Autodesk Inventor part; units mm, degrees
(part 2 of 7)
  line L845 (-272.2013, -12.84) -> (-271.8153, -13.0066)
  line L846 (-271.8153, -13.0066) -> (-271.4089, -13.1307)
  line L847 (-271.4089, -13.1307) -> (-270.9874, -13.2134)
  line L848 (-270.9874, -13.2134) -> (-270.5558, -13.2559)
  line L849 (-270.5558, -13.2559) -> (-270.1196, -13.2593)
  line L850 (-270.1196, -13.2593) -> (-269.6838, -13.2245)
  line L851 (-269.6838, -13.2245) -> (-269.2538, -13.1528)
  line L852 (-269.2538, -13.1528) -> (-268.8348, -13.0453)
  line L853 (-268.8348, -13.0453) -> (-268.4319, -12.9031)
  line L854 (-268.4319, -12.9031) -> (-268.0504, -12.7271)
  line L855 (-268.0504, -12.7271) -> (-267.6956, -12.5187)
  line L856 (-267.6956, -12.5187) -> (-267.3727, -12.2788)
  line L857 (-267.3727, -12.2788) -> (-267.0868, -12.0086)
  line L858 (-267.0868, -12.0086) -> (-266.8433, -11.7091)
  line L859 (-266.8433, -11.7091) -> (-266.6473, -11.3815)
  line L860 (-266.6473, -11.3815) -> (-266.462, -10.9873)
  line L861 (-266.462, -10.9873) -> (-266.3277, -10.6383)
  line L862 (-266.3277, -10.6383) -> (-266.2438, -10.3185)
  line L863 (-266.2438, -10.3185) -> (-266.2099, -10.0121)
  line L864 (-266.2099, -10.0121) -> (-266.2256, -9.703)
  line L865 (-266.2256, -9.703) -> (-266.2902, -9.3753)
  line L866 (-266.2902, -9.3753) -> (-266.4035, -9.013)
  line L867 (-266.4035, -9.013) -> (-266.5648, -8.6003)
  line L868 (-267.3452, -32.2865) -> (-267.8792, -32.2536)
  line L869 (-267.8792, -32.2536) -> (-268.3624, -32.1575)
  line L870 (-268.3624, -32.1575) -> (-268.7797, -32.0027)
  line L871 (-268.7797, -32.0027) -> (-269.116, -31.7932)
  line L872 (-269.116, -31.7932) -> (-269.7252, -31.2998)
  line L873 (-269.7252, -31.2998) -> (-267.9545, -30.2814)
  line L874 (-267.9545, -30.2814) -> (-267.6846, -30.1248)
  line L875 (-267.6846, -30.1248) -> (-267.4428, -29.9813)
  line L876 (-267.4428, -29.9813) -> (-267.2276, -29.8494)
  line L877 (-267.2276, -29.8494) -> (-267.0377, -29.7277)
  line L878 (-267.0377, -29.7277) -> (-266.7274, -29.5089)
  line L879 (-266.7274, -29.5089) -> (-266.5001, -29.3132)
  line L880 (-266.5001, -29.3132) -> (-266.3439, -29.1287)
  line L881 (-266.3439, -29.1287) -> (-266.2471, -28.9437)
  line L882 (-266.2471, -28.9437) -> (-266.1976, -28.7466)
  line L883 (-266.1976, -28.7466) -> (-266.1838, -28.5255)
  line L884 (-266.1838, -28.5255) -> (-266.1936, -28.2391)
  line L885 (-266.1936, -28.2391) -> (-266.2202, -28.0046)
  line L886 (-266.2202, -28.0046) -> (-266.2386, -27.9144)
  line L887 (-266.2386, -27.9144) -> (-266.2597, -27.8462)
  line L888 (-266.2597, -27.8462) -> (-266.283, -27.803)
  line L889 (-266.283, -27.803) -> (-266.308, -27.788)
  line L890 (-266.308, -27.788) -> (-266.379, -27.8152)
  line L891 (-266.379, -27.8152) -> (-266.5342, -27.8931)
  line L892 (-266.5342, -27.8931) -> (-266.7639, -28.0164)
  line L893 (-266.7639, -28.0164) -> (-267.0584, -28.1794)
  line L894 (-267.0584, -28.1794) -> (-267.4079, -28.3768)
  line L895 (-267.4079, -28.3768) -> (-267.8025, -28.6032)
  line L896 (-267.8025, -28.6032) -> (-268.2326, -28.8529)
  line L897 (-268.2326, -28.8529) -> (-268.6883, -29.1206)
  line L898 (-268.6883, -29.1206) -> (-270.9445, -30.4532)
  line L899 (-270.9445, -30.4532) -> (-272.359, -29.3852)
  line L900 (-272.359, -29.3852) -> (-272.6467, -29.1707)
  line L901 (-272.6467, -29.1707) -> (-272.922, -28.9705)
  line L902 (-272.922, -28.9705) -> (-273.1783, -28.7891)
  line L903 (-273.1783, -28.7891) -> (-273.4093, -28.6309)
  line L904 (-273.4093, -28.6309) -> (-273.6082, -28.5003)
  line L905 (-273.6082, -28.5003) -> (-273.7686, -28.4015)
  line L906 (-273.7686, -28.4015) -> (-273.884, -28.339)
  line L907 (-273.884, -28.339) -> (-273.948, -28.3172)
  line L908 (-273.948, -28.3172) -> (-274.0152, -28.3746)
  line L909 (-274.0152, -28.3746) -> (-274.0693, -28.531)
  line L910 (-274.0693, -28.531) -> (-274.1047, -28.7624)
  line L911 (-274.1047, -28.7624) -> (-274.116, -29.0449)
  line L912 (-274.116, -29.0449) -> (-274.099, -29.2561)
  line L913 (-274.099, -29.2561) -> (-274.0465, -29.4524)
  line L914 (-274.0465, -29.4524) -> (-273.9505, -29.6431)
  line L915 (-273.9505, -29.6431) -> (-273.8029, -29.8373)
  line L916 (-273.8029, -29.8373) -> (-273.5956, -30.0441)
  line L917 (-273.5956, -30.0441) -> (-273.3205, -30.2725)
  line L918 (-273.3205, -30.2725) -> (-272.9695, -30.5318)
  line L919 (-272.9695, -30.5318) -> (-272.5347, -30.8311)
  line L920 (-272.5347, -30.8311) -> (-272.2182, -31.0478)
  line L921 (-272.2182, -31.0478) -> (-271.9226, -31.2577)
  line L922 (-271.9226, -31.2577) -> (-271.6546, -31.4559)
  line L923 (-271.6546, -31.4559) -> (-271.4205, -31.6369)
  line L924 (-271.4205, -31.6369) -> (-271.2268, -31.7959)
  line L925 (-271.2268, -31.7959) -> (-271.0801, -31.9275)
  line L926 (-271.0801, -31.9275) -> (-270.9867, -32.0266)
  line L927 (-270.9867, -32.0266) -> (-270.9533, -32.088)
  line L928 (-270.9533, -32.088) -> (-270.9845, -32.1279)
  line L929 (-270.9845, -32.1279) -> (-271.0761, -32.1651)
  line L930 (-271.0761, -32.1651) -> (-271.2219, -32.1988)
  line L931 (-271.2219, -32.1988) -> (-271.4152, -32.2282)
  line L932 (-271.4152, -32.2282) -> (-271.6496, -32.2525)
  line L933 (-271.6496, -32.2525) -> (-271.9187, -32.2708)
  line L934 (-271.9187, -32.2708) -> (-272.2158, -32.2825)
  line L935 (-272.2158, -32.2825) -> (-272.5347, -32.2865)
  line L936 (-272.5347, -32.2865) -> (-274.1224, -32.2865)
  line L937 (-274.1224, -32.2865) -> (-274.1224, -33.0804)
  line L938 (-274.1224, -33.0804) -> (-274.1224, -33.8742)
  line L939 (-274.1224, -33.8742) -> (-270.1531, -33.8742)
  line L940 (-270.1531, -33.8742) -> (-266.1838, -33.8742)
  line L941 (-266.1838, -33.8742) -> (-266.1838, -33.0804)
  line L942 (-266.1838, -33.0804) -> (-266.188, -32.8276)
  line L943 (-266.188, -32.8276) -> (-266.2086, -32.6351)
  line L944 (-266.2086, -32.6351) -> (-266.2575, -32.4945)
  line L945 (-266.2575, -32.4945) -> (-266.3467, -32.3979)
  line L946 (-266.3467, -32.3979) -> (-266.4881, -32.3369)
  line L947 (-266.4881, -32.3369) -> (-266.6937, -32.3035)
  line L948 (-266.6937, -32.3035) -> (-266.9755, -32.2894)
  line L949 (-266.9755, -32.2894) -> (-267.3452, -32.2865)
  line L950 (-270.1531, 32.2808) -> (-274.1224, 32.2808)
  line L951 (-274.1224, 32.2808) -> (-274.1224, 31.6192)
  line L952 (-274.1224, 31.6192) -> (-274.1224, 30.9577)
  line L953 (-274.1224, 30.9577) -> (-270.1531, 30.9577)
  line L954 (-270.1531, 30.9577) -> (-266.1838, 30.9577)
  line L955 (-266.1838, 30.9577) -> (-266.1838, 31.6192)
  line L956 (-266.1838, 31.6192) -> (-266.1838, 32.2808)
  line L957 (-266.1838, 32.2808) -> (-270.1531, 32.2808)
  line L958 (-267.6392, -18.7909) -> (-267.8826, -18.7903)
  line L959 (-267.8826, -18.7903) -> (-268.0973, -18.7881)
  line L960 (-268.0973, -18.7881) -> (-268.2851, -18.7835)
  line L961 (-268.2851, -18.7835) -> (-268.4478, -18.7755)
  line L962 (-268.4478, -18.7755) -> (-268.7051, -18.7465)
  line L963 (-268.7051, -18.7465) -> (-268.8835, -18.6945)
  line L964 (-268.8835, -18.6945) -> (-268.9974, -18.6131)
  line L965 (-268.9974, -18.6131) -> (-269.0609, -18.4956)
  line L966 (-269.0609, -18.4956) -> (-269.0886, -18.3356)
  line L967 (-269.0886, -18.3356) -> (-269.0946, -18.1265)
  line L968 (-269.0946, -18.1265) -> (-269.0808, -17.9354)
  line L969 (-269.0808, -17.9354) -> (-269.0343, -17.7642)
  line L970 (-269.0343, -17.7642) -> (-268.9474, -17.6057)
  line L971 (-268.9474, -17.6057) -> (-268.8125, -17.4525)
  line L972 (-268.8125, -17.4525) -> (-268.6218, -17.2974)
  line L973 (-268.6218, -17.2974) -> (-268.3679, -17.1332)
  line L974 (-268.3679, -17.1332) -> (-268.0429, -16.9525)
  line L975 (-268.0429, -16.9525) -> (-267.6392, -16.7482)
  line L976 (-267.6392, -16.7482) -> (-267.4074, -16.6334)
  line L977 (-267.4074, -16.6334) -> (-267.2014, -16.5284)
  line L978 (-267.2014, -16.5284) -> (-267.0195, -16.4315)
  line L979 (-267.0195, -16.4315) -> (-266.8603, -16.3412)
  line L980 (-266.8603, -16.3412) -> (-266.6043, -16.174)
  line L981 (-266.6043, -16.174) -> (-266.4213, -16.0143)
  line L982 (-266.4213, -16.0143) -> (-266.2996, -15.8493)
  line L983 (-266.2996, -15.8493) -> (-266.2274, -15.6666)
  line L984 (-266.2274, -15.6666) -> (-266.1927, -15.4534)
  line L985 (-266.1927, -15.4534) -> (-266.1838, -15.1971)
  line L986 (-266.1838, -15.1971) -> (-266.1838, -14.3597)
  line L987 (-266.1838, -14.3597) -> (-267.7535, -15.1829)
  line L988 (-267.7535, -15.1829) -> (-269.3232, -16.0061)
  line L989 (-269.3232, -16.0061) -> (-269.9537, -15.4139)
  line L990 (-269.9537, -15.4139) -> (-270.247, -15.1962)
  line L991 (-270.247, -15.1962) -> (-270.6031, -15.0254)
  line L992 (-270.6031, -15.0254) -> (-271.0044, -14.9035)
  line L993 (-271.0044, -14.9035) -> (-271.4332, -14.8321)
  line L994 (-271.4332, -14.8321) -> (-271.8718, -14.8131)
  line L995 (-271.8718, -14.8131) -> (-272.3025, -14.8485)
  line L996 (-272.3025, -14.8485) -> (-272.7077, -14.9399)
  line L997 (-272.7077, -14.9399) -> (-273.0697, -15.0893)
  line L998 (-273.0697, -15.0893) -> (-273.1839, -15.1649)
  line L999 (-273.1839, -15.1649) -> (-273.2933, -15.2662)
  line L1000 (-273.2933, -15.2662) -> (-273.3974, -15.3921)
  line L1001 (-273.3974, -15.3921) -> (-273.496, -15.5412)
  line L1002 (-273.496, -15.5412) -> (-273.675, -15.9049)
  line L1003 (-273.675, -15.9049) -> (-273.8277, -16.3478)
  line L1004 (-273.8277, -16.3478) -> (-273.9514, -16.8606)
  line L1005 (-273.9514, -16.8606) -> (-274.0433, -17.434)
  line L1006 (-274.0433, -17.434) -> (-274.1007, -18.0585)
  line L1007 (-274.1007, -18.0585) -> (-274.1209, -18.7247)
  line L1008 (-274.1209, -18.7247) -> (-274.1224, -20.114)
  line L1009 (-274.1224, -20.114) -> (-270.1531, -20.114)
  line L1010 (-270.1531, -20.114) -> (-266.1838, -20.114)
  line L1011 (-266.1838, -20.114) -> (-266.1838, -19.4524)
  line L1012 (-266.1838, -19.4524) -> (-266.1899, -19.2444)
  line L1013 (-266.1899, -19.2444) -> (-266.2177, -19.0852)
  line L1014 (-266.2177, -19.0852) -> (-266.2814, -18.9683)
  line L1015 (-266.2814, -18.9683) -> (-266.3955, -18.8871)
  line L1016 (-266.3955, -18.8871) -> (-266.574, -18.8353)
  line L1017 (-266.574, -18.8353) -> (-266.8313, -18.8063)
  line L1018 (-266.8313, -18.8063) -> (-266.9939, -18.7983)
  line L1019 (-266.9939, -18.7983) -> (-267.1816, -18.7937)
  line L1020 (-267.1816, -18.7937) -> (-267.3961, -18.7914)
  line L1021 (-267.3961, -18.7914) -> (-267.6392, -18.7909)
  line L1022 (-266.9776, 6.348) -> (-267.7715, 6.348)
  line L1023 (-267.7715, 6.348) -> (-267.7715, 4.628)
  line L1024 (-267.7715, 4.628) -> (-267.7715, 2.9079)
  line L1025 (-267.7715, 2.9079) -> (-268.6977, 2.9079)
  line L1026 (-268.6977, 2.9079) -> (-269.6238, 2.9079)
  line L1027 (-269.6238, 2.9079) -> (-269.6238, 4.2311)
  line L1028 (-269.6238, 4.2311) -> (-269.6269, 4.6425)
  line L1029 (-269.6269, 4.6425) -> (-269.6404, 4.9588)
  line L1030 (-269.6404, 4.9588) -> (-269.6703, 5.1924)
  line L1031 (-269.6703, 5.1924) -> (-269.7231, 5.3557)
  line L1032 (-269.7231, 5.3557) -> (-269.8047, 5.4611)
  line L1033 (-269.8047, 5.4611) -> (-269.9215, 5.5211)
  line L1034 (-269.9215, 5.5211) -> (-270.0797, 5.5479)
  line L1035 (-270.0797, 5.5479) -> (-270.2854, 5.5542)
  line L1036 (-270.2854, 5.5542) -> (-270.4911, 5.5479)
  line L1037 (-270.4911, 5.5479) -> (-270.6492, 5.5211)
  line L1038 (-270.6492, 5.5211) -> (-270.766, 5.4611)
  line L1039 (-270.766, 5.4611) -> (-270.8477, 5.3557)
  line L1040 (-270.8477, 5.3557) -> (-270.9004, 5.1924)
  line L1041 (-270.9004, 5.1924) -> (-270.9304, 4.9588)
  line L1042 (-270.9304, 4.9588) -> (-270.9438, 4.6425)
  line L1043 (-270.9438, 4.6425) -> (-270.9469, 4.2311)
  line L1044 (-270.9469, 4.2311) -> (-270.9473, 4.003)
  line L1045 (-270.9473, 4.003) -> (-270.9492, 3.8028)
  line L1046 (-270.9492, 3.8028) -> (-270.9537, 3.6285)
  line L1047 (-270.9537, 3.6285) -> (-270.9618, 3.4785)
  line L1048 (-270.9618, 3.4785) -> (-270.9935, 3.2439)
  line L1049 (-270.9935, 3.2439) -> (-271.0528, 3.0844)
  line L1050 (-271.0528, 3.0844) -> (-271.1485, 2.9855)
  line L1051 (-271.1485, 2.9855) -> (-271.2893, 2.9328)
  line L1052 (-271.2893, 2.9328) -> (-271.4838, 2.9117)
  line L1053 (-271.4838, 2.9117) -> (-271.7408, 2.9079)
  line L1054 (-271.7408, 2.9079) -> (-272.5347, 2.9079)
  line L1055 (-272.5347, 2.9079) -> (-272.5347, 4.4957)
  line L1056 (-272.5347, 4.4957) -> (-272.5347, 6.0834)
  line L1057 (-272.5347, 6.0834) -> (-273.3285, 6.0834)
  line L1058 (-273.3285, 6.0834) -> (-274.1224, 6.0834)
  line L1059 (-274.1224, 6.0834) -> (-274.1224, 3.8341)
  line L1060 (-274.1224, 3.8341) -> (-274.1224, 1.5849)
  line L1061 (-274.1224, 1.5849) -> (-270.1531, 1.5849)
  line L1062 (-270.1531, 1.5849) -> (-266.1838, 1.5849)
  line L1063 (-266.1838, 1.5849) -> (-266.1838, 3.9664)
  line L1064 (-266.1838, 3.9664) -> (-266.1838, 6.348)
  line L1065 (-266.1838, 6.348) -> (-266.9776, 6.348)
  line L1066 (-271.4762, -18.7909) -> (-272.5651, -18.7909)
  line L1067 (-272.5651, -18.7909) -> (-272.4837, -17.6932)
  line L1068 (-272.4837, -17.6932) -> (-272.4371, -17.3233)
  line L1069 (-272.4371, -17.3233) -> (-272.3587, -17.0028)
  line L1070 (-272.3587, -17.0028) -> (-272.2532, -16.7315)
  line L1071 (-272.2532, -16.7315) -> (-272.125, -16.5096)
  line L1072 (-272.125, -16.5096) -> (-271.9786, -16.337)
  line L1073 (-271.9786, -16.337) -> (-271.8187, -16.2137)
  line L1074 (-271.8187, -16.2137) -> (-271.6497, -16.1397)
  line L1075 (-271.6497, -16.1397) -> (-271.4762, -16.1151)
  line L1076 (-271.4762, -16.1151) -> (-271.3026, -16.1397)
  line L1077 (-271.3026, -16.1397) -> (-271.1336, -16.2137)
  line L1078 (-271.1336, -16.2137) -> (-270.9737, -16.337)
  line L1079 (-270.9737, -16.337) -> (-270.8273, -16.5096)
  line L1080 (-270.8273, -16.5096) -> (-270.6991, -16.7315)
  line L1081 (-270.6991, -16.7315) -> (-270.5936, -17.0028)
  line L1082 (-270.5936, -17.0028) -> (-270.5152, -17.3233)
  line L1083 (-270.5152, -17.3233) -> (-270.4686, -17.6932)
  line L1084 (-270.4686, -17.6932) -> (-270.3873, -18.7909)
  line L1085 (-270.3873, -18.7909) -> (-271.4762, -18.7909)
  line L1086 (-269.3592, -23.8187) -> (-272.5347, -23.8187)
  line L1087 (-272.5347, -23.8187) -> (-272.5347, -22.7602)
  line L1088 (-272.5347, -22.7602) -> (-272.538, -22.4277)
  line L1089 (-272.538, -22.4277) -> (-272.5533, -22.1731)
  line L1090 (-272.5533, -22.1731) -> (-272.5882, -21.986)
  line L1091 (-272.5882, -21.986) -> (-272.6504, -21.8561)
  line L1092 (-272.6504, -21.8561) -> (-272.7478, -21.773)
  line L1093 (-272.7478, -21.773) -> (-272.8882, -21.7265)
  line L1094 (-272.8882, -21.7265) -> (-273.0791, -21.7062)
  line L1095 (-273.0791, -21.7062) -> (-273.3285, -21.7017)
  line L1096 (-273.3285, -21.7017) -> (-274.1224, -21.7017)
  line L1097 (-274.1224, -21.7017) -> (-274.1224, -24.6125)
  line L1098 (-274.1224, -24.6125) -> (-274.1224, -27.5233)
  line L1099 (-274.1224, -27.5233) -> (-273.3285, -27.5233)
  line L1100 (-273.3285, -27.5233) -> (-273.0791, -27.5189)
  line L1101 (-273.0791, -27.5189) -> (-272.8882, -27.4985)
  line L1102 (-272.8882, -27.4985) -> (-272.7478, -27.452)
  line L1103 (-272.7478, -27.452) -> (-272.6504, -27.369)
  line L1104 (-272.6504, -27.369) -> (-272.5882, -27.2391)
  line L1105 (-272.5882, -27.2391) -> (-272.5533, -27.052)
  line L1106 (-272.5533, -27.052) -> (-272.538, -26.7974)
  line L1107 (-272.538, -26.7974) -> (-272.5347, -26.4649)
  line L1108 (-272.5347, -26.4649) -> (-272.5347, -25.4064)
  line L1109 (-272.5347, -25.4064) -> (-269.3592, -25.4064)
  line L1110 (-269.3592, -25.4064) -> (-266.1838, -25.4064)
  line L1111 (-266.1838, -25.4064) -> (-266.1838, -24.6125)
  line L1112 (-266.1838, -24.6125) -> (-266.1838, -23.8187)
  line L1113 (-266.1838, -23.8187) -> (-269.3592, -23.8187)
  line L1114 (-267.2516, 35.9855) -> (-267.6695, 36.0151)
  line L1115 (-267.6695, 36.0151) -> (-268.0934, 36.0965)
  line L1116 (-268.0934, 36.0965) -> (-268.5004, 36.2188)
  line L1117 (-268.5004, 36.2188) -> (-268.8676, 36.3711)
  line L1118 (-268.8676, 36.3711) -> (-269.1723, 36.5421)
  line L1119 (-269.1723, 36.5421) -> (-269.3916, 36.7211)
  line L1120 (-269.3916, 36.7211) -> (-269.462, 36.8101)
  line L1121 (-269.462, 36.8101) -> (-269.5025, 36.897)
  line L1122 (-269.5025, 36.897) -> (-269.5103, 36.9803)
  line L1123 (-269.5103, 36.9803) -> (-269.4824, 37.0588)
  line L1124 (-269.4824, 37.0588) -> (-269.4226, 37.121)
  line L1125 (-269.4226, 37.121) -> (-269.3045, 37.2133)
  line L1126 (-269.3045, 37.2133) -> (-269.135, 37.3313)
  line L1127 (-269.135, 37.3313) -> (-268.9213, 37.4705)
  line L1128 (-268.9213, 37.4705) -> (-268.3892, 37.7944)
  line L1129 (-268.3892, 37.7944) -> (-267.7646, 38.1494)
  line L1130 (-267.7646, 38.1494) -> (-267.3115, 38.4045)
  line L1131 (-267.3115, 38.4045) -> (-266.9516, 38.6234)
  line L1132 (-266.9516, 38.6234) -> (-266.6749, 38.8163)
  line L1133 (-266.6749, 38.8163) -> (-266.4711, 38.9937)
  line L1134 (-266.4711, 38.9937) -> (-266.3302, 39.1656)
  line L1135 (-266.3302, 39.1656) -> (-266.2421, 39.3423)
  line L1136 (-266.2421, 39.3423) -> (-266.1967, 39.5341)
  line L1137 (-266.1967, 39.5341) -> (-266.1838, 39.7512)
  line L1138 (-266.1838, 39.7512) -> (-266.1963, 40.0357)
  line L1139 (-266.1963, 40.0357) -> (-266.2303, 40.2687)
  line L1140 (-266.2303, 40.2687) -> (-266.2538, 40.3584)
  line L1141 (-266.2538, 40.3584) -> (-266.2807, 40.4262)
  line L1142 (-266.2807, 40.4262) -> (-266.3104, 40.469)
  line L1143 (-266.3104, 40.469) -> (-266.3422, 40.484)
  line L1144 (-266.3422, 40.484) -> (-266.4193, 40.4574)
  line L1145 (-266.4193, 40.4574) -> (-266.5788, 40.381)
  line L1146 (-266.5788, 40.381) -> (-266.8108, 40.2603)
  line L1147 (-266.8108, 40.2603) -> (-267.1057, 40.1005)
  line L1148 (-267.1057, 40.1005) -> (-267.4536, 39.9071)
  line L1149 (-267.4536, 39.9071) -> (-267.845, 39.6854)
  line L1150 (-267.845, 39.6854) -> (-268.2699, 39.4408)
  line L1151 (-268.2699, 39.4408) -> (-268.7187, 39.1785)
  line L1152 (-268.7187, 39.1785) -> (-270.9367, 37.8731)
  line L1153 (-270.9367, 37.8731) -> (-272.5295, 39.0457)
  line L1154 (-272.5295, 39.0457) -> (-274.1224, 40.2183)
  line L1155 (-274.1224, 40.2183) -> (-274.1224, 39.4243)
  line L1156 (-274.1224, 39.4243) -> (-274.109, 39.1889)
  line L1157 (-274.109, 39.1889) -> (-274.0625, 38.9758)
  line L1158 (-274.0625, 38.9758) -> (-273.973, 38.7732)
  line L1159 (-273.973, 38.7732) -> (-273.8309, 38.5695)
  line L1160 (-273.8309, 38.5695) -> (-273.6264, 38.3527)
  line L1161 (-273.6264, 38.3527) -> (-273.3499, 38.1111)
  line L1162 (-273.3499, 38.1111) -> (-273.1815, 37.9773)
  line L1163 (-273.1815, 37.9773) -> (-272.9915, 37.8329)
  line L1164 (-272.9915, 37.8329) -> (-272.7787, 37.6764)
  line L1165 (-272.7787, 37.6764) -> (-272.5417, 37.5064)
  line L1166 (-272.5417, 37.5064) -> (-272.224, 37.2765)
  line L1167 (-272.224, 37.2765) -> (-271.9274, 37.0543)
  line L1168 (-271.9274, 37.0543) -> (-271.6583, 36.8451)
  line L1169 (-271.6583, 36.8451) -> (-271.4233, 36.6543)
  line L1170 (-271.4233, 36.6543) -> (-271.2288, 36.4873)
  line L1171 (-271.2288, 36.4873) -> (-271.0814, 36.3497)
  line L1172 (-271.0814, 36.3497) -> (-270.9877, 36.2467)
  line L1173 (-270.9877, 36.2467) -> (-270.954, 36.1839)
  line L1174 (-270.954, 36.1839) -> (-270.985, 36.1441)
  line L1175 (-270.985, 36.1441) -> (-271.0765, 36.1069)
  line L1176 (-271.0765, 36.1069) -> (-271.2222, 36.0732)
  line L1177 (-271.2222, 36.0732) -> (-271.4154, 36.0438)
  line L1178 (-271.4154, 36.0438) -> (-271.6497, 36.0195)
  line L1179 (-271.6497, 36.0195) -> (-271.9187, 36.0011)
  line L1180 (-271.9187, 36.0011) -> (-272.2159, 35.9895)
  line L1181 (-272.2159, 35.9895) -> (-272.5347, 35.9855)
  line L1182 (-272.5347, 35.9855) -> (-274.1224, 35.9855)
  line L1183 (-274.1224, 35.9855) -> (-274.1224, 35.1916)
  line L1184 (-274.1224, 35.1916) -> (-274.1224, 34.3977)
  line L1185 (-274.1224, 34.3977) -> (-270.1531, 34.3977)
  line L1186 (-270.1531, 34.3977) -> (-266.1838, 34.3977)
  line L1187 (-266.1838, 34.3977) -> (-266.1838, 35.1916)
  line L1188 (-266.1838, 35.1916) -> (-266.1882, 35.4413)
  line L1189 (-266.1882, 35.4413) -> (-266.2086, 35.6324)
  line L1190 (-266.2086, 35.6324) -> (-266.2553, 35.7728)
  line L1191 (-266.2553, 35.7728) -> (-266.3389, 35.8701)
  line L1192 (-266.3389, 35.8701) -> (-266.4698, 35.9323)
  line L1193 (-266.4698, 35.9323) -> (-266.6586, 35.967)
  line L1194 (-266.6586, 35.967) -> (-266.9157, 35.9822)
  line L1195 (-266.9157, 35.9822) -> (-267.2516, 35.9855)
  line L1196 (-268.9628, 24.2931) -> (-269.5211, 24.2796)
  line L1197 (-269.5211, 24.2796) -> (-270.0419, 24.2734)
  line L1198 (-270.0419, 24.2734) -> (-270.5137, 24.274)
  line L1199 (-270.5137, 24.274) -> (-270.9254, 24.2813)
  line L1200 (-270.9254, 24.2813) -> (-271.2654, 24.2948)
  line L1201 (-271.2654, 24.2948) -> (-271.5223, 24.3143)
  line L1202 (-271.5223, 24.3143) -> (-271.616, 24.3262)
  line L1203 (-271.616, 24.3262) -> (-271.6847, 24.3394)
  line L1204 (-271.6847, 24.3394) -> (-271.727, 24.354)
  line L1205 (-271.727, 24.354) -> (-271.7413, 24.3698)
  line L1206 (-271.7413, 24.3698) -> (-271.7269, 24.3931)
  line L1207 (-271.7269, 24.3931) -> (-271.6845, 24.4296)
  line L1208 (-271.6845, 24.4296) -> (-271.6157, 24.4783)
  line L1209 (-271.6157, 24.4783) -> (-271.5219, 24.5386)
  line L1210 (-271.5219, 24.5386) -> (-271.2648, 24.6907)
  line L1211 (-271.2648, 24.6907) -> (-270.9248, 24.8797)
  line L1212 (-270.9248, 24.8797) -> (-270.5131, 25.0994)
  line L1213 (-270.5131, 25.0994) -> (-270.0412, 25.3436)
  line L1214 (-270.0412, 25.3436) -> (-269.5204, 25.6061)
  line L1215 (-269.5204, 25.6061) -> (-268.9623, 25.8807)
  line L1216 (-268.9623, 25.8807) -> (-268.4989, 26.1067)
  line L1217 (-268.4989, 26.1067) -> (-268.0899, 26.3083)
  line L1218 (-268.0899, 26.3083) -> (-267.7319, 26.4881)
  line L1219 (-267.7319, 26.4881) -> (-267.4216, 26.6487)
  line L1220 (-267.4216, 26.6487) -> (-267.1557, 26.7927)
  line L1221 (-267.1557, 26.7927) -> (-266.9305, 26.9229)
  line L1222 (-266.9305, 26.9229) -> (-266.743, 27.0417)
  line L1223 (-266.743, 27.0417) -> (-266.5895, 27.1519)
  line L1224 (-266.5895, 27.1519) -> (-266.3714, 27.3567)
  line L1225 (-266.3714, 27.3567) -> (-266.2491, 27.5583)
  line L1226 (-266.2491, 27.5583) -> (-266.1956, 27.7778)
  line L1227 (-266.1956, 27.7778) -> (-266.1838, 28.0362)
  line L1228 (-266.1838, 28.0362) -> (-266.1838, 28.8407)
  line L1229 (-266.1838, 28.8407) -> (-270.1531, 28.8407)
  line L1230 (-270.1531, 28.8407) -> (-274.1224, 28.8407)
  line L1231 (-274.1224, 28.8407) -> (-274.1224, 28.1792)
  line L1232 (-274.1224, 28.1792) -> (-274.1224, 27.5176)
  line L1233 (-274.1224, 27.5176) -> (-271.1454, 27.5148)
  line L1234 (-271.1454, 27.5148) -> (-268.1684, 27.512)
  line L1235 (-268.1684, 27.512) -> (-271.1454, 26.0402)
  line L1236 (-271.1454, 26.0402) -> (-271.6369, 25.7964)
  line L1237 (-271.6369, 25.7964) -> (-272.0714, 25.5788)
  line L1238 (-272.0714, 25.5788) -> (-272.4523, 25.3845)
  line L1239 (-272.4523, 25.3845) -> (-272.7832, 25.2111)
  line L1240 (-272.7832, 25.2111) -> (-273.0676, 25.0559)
  line L1241 (-273.0676, 25.0559) -> (-273.3089, 24.9162)
  line L1242 (-273.3089, 24.9162) -> (-273.5106, 24.7894)
  line L1243 (-273.5106, 24.7894) -> (-273.6763, 24.6728)
  line L1244 (-273.6763, 24.6728) -> (-273.8094, 24.5639)
  line L1245 (-273.8094, 24.5639) -> (-273.9134, 24.46)
  line L1246 (-273.9134, 24.46) -> (-273.9918, 24.3585)
  line L1247 (-273.9918, 24.3585) -> (-274.0481, 24.2566)
  line L1248 (-274.0481, 24.2566) -> (-274.1085, 24.0416)
  line L1249 (-274.1085, 24.0416) -> (-274.1224, 23.7937)
  line L1250 (-274.1224, 23.7937) -> (-274.1224, 23.0191)
  line L1251 (-274.1224, 23.0191) -> (-270.1531, 23.0191)
  line L1252 (-270.1531, 23.0191) -> (-266.1838, 23.0191)
  line L1253 (-266.1838, 23.0191) -> (-266.1838, 23.6977)
  line L1254 (-266.1838, 23.6977) -> (-266.1838, 24.3762)
  line L1255 (-266.1838, 24.3762) -> (-268.9628, 24.2931)
  line L1256 (-266.5537, 12.2782) -> (-266.7195, 12.653)
  line L1257 (-266.7195, 12.653) -> (-266.8708, 12.9403)
  line L1258 (-266.8708, 12.9403) -> (-267.0151, 13.1443)
  line L1259 (-267.0151, 13.1443) -> (-267.1598, 13.2696)
  line L1260 (-267.1598, 13.2696) -> (-267.3124, 13.3205)
  line L1261 (-267.3124, 13.3205) -> (-267.4805, 13.3015)
  line L1262 (-267.4805, 13.3015) -> (-267.6713, 13.2169)
  line L1263 (-267.6713, 13.2169) -> (-267.8925, 13.0714)
  line L1264 (-267.8925, 13.0714) -> (-268.0251, 12.9683)
  line L1265 (-268.0251, 12.9683) -> (-268.1253, 12.8753)
  line L1266 (-268.1253, 12.8753) -> (-268.1938, 12.7898)
  line L1267 (-268.1938, 12.7898) -> (-268.2314, 12.709)
  line L1268 (-268.2314, 12.709) -> (-268.2389, 12.6303)
  line L1269 (-268.2389, 12.6303) -> (-268.217, 12.5511)
  line L1270 (-268.217, 12.5511) -> (-268.1665, 12.4687)
  line L1271 (-268.1665, 12.4687) -> (-268.088, 12.3804)
  line L1272 (-268.088, 12.3804) -> (-267.9277, 12.1543)
  line L1273 (-267.9277, 12.1543) -> (-267.8259, 11.8684)
  line L1274 (-267.8259, 11.8684) -> (-267.7811, 11.54)
  line L1275 (-267.7811, 11.54) -> (-267.7913, 11.1865)
  line L1276 (-267.7913, 11.1865) -> (-267.8548, 10.8255)
  line L1277 (-267.8548, 10.8255) -> (-267.9697, 10.4744)
  line L1278 (-267.9697, 10.4744) -> (-268.1344, 10.1505)
  line L1279 (-268.1344, 10.1505) -> (-268.3468, 9.8713)
  line L1280 (-268.3468, 9.8713) -> (-268.5006, 9.7285)
  line L1281 (-268.5006, 9.7285) -> (-268.6748, 9.604)
  line L1282 (-268.6748, 9.604) -> (-268.8669, 9.4978)
  line L1283 (-268.8669, 9.4978) -> (-269.0743, 9.41)
  line L1284 (-269.0743, 9.41) -> (-269.525, 9.2898)
  line L1285 (-269.525, 9.2898) -> (-270.0066, 9.2436)
  line L1286 (-270.0066, 9.2436) -> (-270.4989, 9.2719)
  line L1287 (-270.4989, 9.2719) -> (-270.9817, 9.375)
  line L1288 (-270.9817, 9.375) -> (-271.4346, 9.5534)
  line L1289 (-271.4346, 9.5534) -> (-271.8374, 9.8073)
  line L1290 (-271.8374, 9.8073) -> (-272.0919, 10.0621)
  line L1291 (-272.0919, 10.0621) -> (-272.2942, 10.3738)
  line L1292 (-272.2942, 10.3738) -> (-272.4413, 10.7231)
  line L1293 (-272.4413, 10.7231) -> (-272.5302, 11.0907)
  line L1294 (-272.5302, 11.0907) -> (-272.5577, 11.4573)
  line L1295 (-272.5577, 11.4573) -> (-272.5209, 11.8033)
  line L1296 (-272.5209, 11.8033) -> (-272.4165, 12.1096)
  line L1297 (-272.4165, 12.1096) -> (-272.2416, 12.3568)
  line L1298 (-272.2416, 12.3568) -> (-272.1748, 12.4349)
  line L1299 (-272.1748, 12.4349) -> (-272.1355, 12.5091)
  line L1300 (-272.1355, 12.5091) -> (-272.1243, 12.581)
  line L1301 (-272.1243, 12.581) -> (-272.1419, 12.6517)
  line L1302 (-272.1419, 12.6517) -> (-272.1888, 12.7228)
  line L1303 (-272.1888, 12.7228) -> (-272.2656, 12.7955)
  line L1304 (-272.2656, 12.7955) -> (-272.3731, 12.8712)
  line L1305 (-272.3731, 12.8712) -> (-272.5117, 12.9512)
  line L1306 (-272.5117, 12.9512) -> (-272.7683, 13.0712)
  line L1307 (-272.7683, 13.0712) -> (-272.987, 13.1303)
  line L1308 (-272.987, 13.1303) -> (-273.1745, 13.1235)
  line L1309 (-273.1745, 13.1235) -> (-273.3378, 13.0455)
  line L1310 (-273.3378, 13.0455) -> (-273.4836, 12.8913)
  line L1311 (-273.4836, 12.8913) -> (-273.6188, 12.6557)
  line L1312 (-273.6188, 12.6557) -> (-273.7502, 12.3335)
  line L1313 (-273.7502, 12.3335) -> (-273.8846, 11.9198)
  line L1314 (-273.8846, 11.9198) -> (-273.9688, 11.6175)
  line L1315 (-273.9688, 11.6175) -> (-274.0247, 11.356)
  line L1316 (-274.0247, 11.356) -> (-274.0509, 11.1219)
  line L1317 (-274.0509, 11.1219) -> (-274.0462, 10.9019)
  line L1318 (-274.0462, 10.9019) -> (-274.0094, 10.6828)
  line L1319 (-274.0094, 10.6828) -> (-273.9391, 10.4511)
  line L1320 (-273.9391, 10.4511) -> (-273.8342, 10.1937)
  line L1321 (-273.8342, 10.1937) -> (-273.6934, 9.8972)
  line L1322 (-273.6934, 9.8972) -> (-273.3978, 9.3671)
  line L1323 (-273.3978, 9.3671) -> (-273.0765, 8.9234)
  line L1324 (-273.0765, 8.9234) -> (-272.7213, 8.5612)
  line L1325 (-272.7213, 8.5612) -> (-272.3242, 8.2755)
  line L1326 (-272.3242, 8.2755) -> (-271.8769, 8.0618)
  line L1327 (-271.8769, 8.0618) -> (-271.3714, 7.915)
  line L1328 (-271.3714, 7.915) -> (-270.7995, 7.8305)
  line L1329 (-270.7995, 7.8305) -> (-270.1531, 7.8034)
  line L1330 (-270.1531, 7.8034) -> (-269.5173, 7.8301)
  line L1331 (-269.5173, 7.8301) -> (-268.9518, 7.9129)
  line L1332 (-268.9518, 7.9129) -> (-268.4496, 8.0556)
  line L1333 (-268.4496, 8.0556) -> (-268.0038, 8.2623)
  line L1334 (-268.0038, 8.2623) -> (-267.6076, 8.5368)
  line L1335 (-267.6076, 8.5368) -> (-267.254, 8.8831)
  line L1336 (-267.254, 8.8831) -> (-266.9362, 9.3052)
  line L1337 (-266.9362, 9.3052) -> (-266.6473, 9.8069)
  line L1338 (-266.6473, 9.8069) -> (-266.4632, 10.1814)
  line L1339 (-266.4632, 10.1814) -> (-266.3299, 10.496)
  line L1340 (-266.3299, 10.496) -> (-266.2467, 10.7712)
  line L1341 (-266.2467, 10.7712) -> (-266.2127, 11.0278)
  line L1342 (-266.2127, 11.0278) -> (-266.2272, 11.2861)
  line L1343 (-266.2272, 11.2861) -> (-266.2894, 11.5669)
  line L1344 (-266.2894, 11.5669) -> (-266.3985, 11.8907)
  line L1345 (-266.3985, 11.8907) -> (-266.5537, 12.2782)
  line L1346 (-269.3592, -2.1198) -> (-272.5347, -2.1198)
  line L1347 (-272.5347, -2.1198) -> (-272.5347, -1.0613)
  line L1348 (-272.5347, -1.0613) -> (-272.538, -0.7288)
  line L1349 (-272.538, -0.7288) -> (-272.5533, -0.4742)
  line L1350 (-272.5533, -0.4742) -> (-272.5882, -0.2871)
  line L1351 (-272.5882, -0.2871) -> (-272.6504, -0.1572)
  line L1352 (-272.6504, -0.1572) -> (-272.7478, -0.0742)
  line L1353 (-272.7478, -0.0742) -> (-272.8882, -0.0277)
  line L1354 (-272.8882, -0.0277) -> (-273.0791, -0.0073)
  line L1355 (-273.0791, -0.0073) -> (-273.3285, -0.0029)
  line L1356 (-273.3285, -0.0029) -> (-274.1224, -0.0029)
  line L1357 (-274.1224, -0.0029) -> (-274.1224, -2.9137)
  line L1358 (-274.1224, -2.9137) -> (-274.1224, -5.8245)
  line L1359 (-274.1224, -5.8245) -> (-273.3285, -5.8245)
  line L1360 (-273.3285, -5.8245) -> (-273.0791, -5.82)
  line L1361 (-273.0791, -5.82) -> (-272.8882, -5.7997)
  line L1362 (-272.8882, -5.7997) -> (-272.7478, -5.7532)
  line L1363 (-272.7478, -5.7532) -> (-272.6504, -5.6701)
  line L1364 (-272.6504, -5.6701) -> (-272.5882, -5.5402)
  line L1365 (-272.5882, -5.5402) -> (-272.5533, -5.3532)
  line L1366 (-272.5533, -5.3532) -> (-272.538, -5.0985)
  line L1367 (-272.538, -5.0985) -> (-272.5347, -4.766)
  line L1368 (-272.5347, -4.766) -> (-272.5347, -3.7075)
  line L1369 (-272.5347, -3.7075) -> (-269.3592, -3.7075)
  line L1370 (-269.3592, -3.7075) -> (-266.1838, -3.7075)
  line L1371 (-266.1838, -3.7075) -> (-266.1838, -2.9137)
  line L1372 (-266.1838, -2.9137) -> (-266.1838, -2.1198)
  line L1373 (-266.1838, -2.1198) -> (-269.3592, -2.1198)
  line L1374 (-267.9038, 16.4036) -> (-269.6238, 16.4036)
  line L1375 (-269.6238, 16.4036) -> (-269.6238, 17.859)
  line L1376 (-269.6238, 17.859) -> (-269.6238, 19.3144)
  line L1377 (-269.6238, 19.3144) -> (-267.9038, 19.3144)
  line L1378 (-267.9038, 19.3144) -> (-266.1838, 19.3144)
  line L1379 (-266.1838, 19.3144) -> (-266.1838, 20.1083)
  line L1380 (-266.1838, 20.1083) -> (-266.1838, 20.9021)
  line L1381 (-266.1838, 20.9021) -> (-270.1531, 20.9021)
  line L1382 (-270.1531, 20.9021) -> (-274.1224, 20.9021)
  line L1383 (-274.1224, 20.9021) -> (-274.1224, 20.1083)
  line L1384 (-274.1224, 20.1083) -> (-274.1189, 19.8485)
  line L1385 (-274.1189, 19.8485) -> (-274.0975, 19.6527)
  line L1386 (-274.0975, 19.6527) -> (-274.0417, 19.5117)
  line L1387 (-274.0417, 19.5117) -> (-273.9349, 19.4166)
  line L1388 (-273.9349, 19.4166) -> (-273.7606, 19.3584)
  line L1389 (-273.7606, 19.3584) -> (-273.5022, 19.3279)
  line L1390 (-273.5022, 19.3279) -> (-273.3363, 19.3203)
  line L1391 (-273.3363, 19.3203) -> (-273.1431, 19.3163)
  line L1392 (-273.1431, 19.3163) -> (-272.9207, 19.3147)
  line L1393 (-272.9207, 19.3147) -> (-272.667, 19.3144)
  line L1394 (-272.667, 19.3144) -> (-271.2115, 19.3144)
  line L1395 (-271.2115, 19.3144) -> (-271.2115, 17.859)
  line L1396 (-271.2115, 17.859) -> (-271.2115, 16.4036)
  line L1397 (-271.2115, 16.4036) -> (-272.667, 16.4036)
  line L1398 (-272.667, 16.4036) -> (-272.9101, 16.403)
  line L1399 (-272.9101, 16.403) -> (-273.1246, 16.4008)
  line L1400 (-273.1246, 16.4008) -> (-273.3122, 16.3961)
  line L1401 (-273.3122, 16.3961) -> (-273.4749, 16.3882)
  line L1402 (-273.4749, 16.3882) -> (-273.7322, 16.3592)
  line L1403 (-273.7322, 16.3592) -> (-273.9107, 16.3073)
  line L1404 (-273.9107, 16.3073) -> (-274.0247, 16.2262)
  line L1405 (-274.0247, 16.2262) -> (-274.0885, 16.1093)
  line L1406 (-274.0885, 16.1093) -> (-274.1163, 15.95)
  line L1407 (-274.1163, 15.95) -> (-274.1224, 15.742)
  line L1408 (-274.1224, 15.742) -> (-274.1224, 15.0805)
  line L1409 (-274.1224, 15.0805) -> (-270.1531, 15.0805)
  line L1410 (-270.1531, 15.0805) -> (-266.1838, 15.0805)
  line L1411 (-266.1838, 15.0805) -> (-266.1838, 15.742)
  line L1412 (-266.1838, 15.742) -> (-266.1897, 15.9536)
  line L1413 (-266.1897, 15.9536) -> (-266.2193, 16.1145)
  line L1414 (-266.2193, 16.1145) -> (-266.2908, 16.2316)
  line L1415 (-266.2908, 16.2316) -> (-266.4219, 16.312)
  line L1416 (-266.4219, 16.312) -> (-266.6308, 16.3624)
  line L1417 (-266.6308, 16.3624) -> (-266.9355, 16.3899)
  line L1418 (-266.9355, 16.3899) -> (-267.1293, 16.3972)
  line L1419 (-267.1293, 16.3972) -> (-267.3538, 16.4013)
  line L1420 (-267.3538, 16.4013) -> (-267.6112, 16.4032)
  line L1421 (-267.6112, 16.4032) -> (-267.9038, 16.4036)
  line L1422 (-166.0823, 11.7473) -> (-166.0051, 12.144)
  line L1423 (-166.0051, 12.144) -> (-165.8608, 12.5181)
  line L1424 (-165.8608, 12.5181) -> (-165.6534, 12.8614)
  line L1425 (-165.6534, 12.8614) -> (-165.387, 13.1653)
  line L1426 (-165.387, 13.1653) -> (-165.1683, 13.3567)
  line L1427 (-165.1683, 13.3567) -> (-165.9495, 13.3567)
  line L1428 (-165.9495, 13.3567) -> (-165.9495, 14.3723)
  line L1429 (-165.9495, 14.3723) -> (-160.3479, 14.3723)
  line L1430 (-160.3479, 14.3723) -> (-159.9593, 14.3708)
  line L1431 (-159.9593, 14.3708) -> (-159.5715, 14.3501)
  line L1432 (-159.5715, 14.3501) -> (-159.1852, 14.3102)
  line L1433 (-159.1852, 14.3102) -> (-158.8011, 14.2512)
  line L1434 (-158.8011, 14.2512) -> (-158.4788, 14.1733)
  line L1435 (-158.4788, 14.1733) -> (-158.1739, 14.048)
  line L1436 (-158.1739, 14.048) -> (-157.8915, 13.8777)
  line L1437 (-157.8915, 13.8777) -> (-157.637, 13.6653)
  line L1438 (-157.637, 13.6653) -> (-157.4026, 13.3997)
  line L1439 (-157.4026, 13.3997) -> (-157.2034, 13.0872)
  line L1440 (-157.2034, 13.0872) -> (-157.0433, 12.7317)
  line L1441 (-157.0433, 12.7317) -> (-156.93, 12.3411)
  line L1442 (-156.93, 12.3411) -> (-156.8597, 11.9114)
  line L1443 (-156.8597, 11.9114) -> (-156.8396, 11.3994)
  line L1444 (-156.8396, 11.3994) -> (-156.8714, 10.8879)
  line L1445 (-156.8714, 10.8879) -> (-156.9294, 10.5365)
  line L1446 (-156.9294, 10.5365) -> (-157.0312, 10.1966)
  line L1447 (-157.0312, 10.1966) -> (-157.1751, 9.8723)
  line L1448 (-157.1751, 9.8723) -> (-157.3597, 9.5676)
  line L1449 (-157.3597, 9.5676) -> (-157.5758, 9.3234)
  line L1450 (-157.5758, 9.3234) -> (-157.8338, 9.1292)
  line L1451 (-157.8338, 9.1292) -> (-158.1253, 8.9902)
  line L1452 (-158.1253, 8.9902) -> (-158.4417, 8.9114)
  line L1453 (-158.4417, 8.9114) -> (-158.6851, 8.8834)
  line L1454 (-158.6851, 8.8834) -> (-158.93, 8.8762)
  line L1455 (-158.93, 8.8762) -> (-158.7737, 9.9465)
  line L1456 (-158.7737, 9.9465) -> (-158.5535, 9.9904)
  line L1457 (-158.5535, 9.9904) -> (-158.344, 10.0715)
  line L1458 (-158.344, 10.0715) -> (-158.1852, 10.1798)
  line L1459 (-158.1852, 10.1798) -> (-158.0511, 10.3176)
  line L1460 (-158.0511, 10.3176) -> (-157.9183, 10.5403)
  line L1461 (-157.9183, 10.5403) -> (-157.8212, 10.8139)
  line L1462 (-157.8212, 10.8139) -> (-157.7659, 11.0989)
  line L1463 (-157.7659, 11.0989) -> (-157.7464, 11.4465)
  line L1464 (-157.7464, 11.4465) -> (-157.7659, 11.7942)
  line L1465 (-157.7659, 11.7942) -> (-157.8203, 12.0947)
  line L1466 (-157.8203, 12.0947) -> (-157.9183, 12.384)
  line L1467 (-157.9183, 12.384) -> (-158.0511, 12.6145)
  line L1468 (-158.0511, 12.6145) -> (-158.2204, 12.8033)
  line L1469 (-158.2204, 12.8033) -> (-158.4183, 12.9622)
  line L1470 (-158.4183, 12.9622) -> (-158.6546, 13.0858)
  line L1471 (-158.6546, 13.0858) -> (-158.9065, 13.1731)
  line L1472 (-158.9065, 13.1731) -> (-159.3656, 13.2342)
  line L1473 (-159.3656, 13.2342) -> (-159.8284, 13.2512)
  line L1474 (-159.8284, 13.2512) -> (-160.0725, 13.2552)
  line L1475 (-160.0725, 13.2552) -> (-160.3167, 13.2551)
  line L1476 (-160.3167, 13.2551) -> (-160.0818, 13.0354)
  line L1477 (-160.0818, 13.0354) -> (-159.8806, 12.7865)
  line L1478 (-159.8806, 12.7865) -> (-159.7159, 12.5121)
  line L1479 (-159.7159, 12.5121) -> (-159.5901, 12.2161)
  line L1480 (-159.5901, 12.2161) -> (-159.4968, 11.8424)
  line L1481 (-159.4968, 11.8424) -> (-159.469, 11.4583)
  line L1482 (-159.469, 11.4583) -> (-159.4742, 11.2251)
  line L1483 (-159.4742, 11.2251) -> (-159.4988, 10.9935)
  line L1484 (-159.4988, 10.9935) -> (-159.5427, 10.7648)
  line L1485 (-159.5427, 10.7648) -> (-159.6058, 10.5403)
  line L1486 (-159.6058, 10.5403) -> (-159.7434, 10.2071)
  line L1487 (-159.7434, 10.2071) -> (-159.9298, 9.9012)
  line L1488 (-159.9298, 9.9012) -> (-160.1613, 9.6276)
  line L1489 (-160.1613, 9.6276) -> (-160.4339, 9.3918)
  line L1490 (-160.4339, 9.3918) -> (-160.8845, 9.102)
  line L1491 (-160.8845, 9.102) -> (-161.3703, 8.883)
  line L1492 (-161.3703, 8.883) -> (-161.883, 8.7377)
  line L1493 (-161.883, 8.7377) -> (-162.4144, 8.6692)
  line L1494 (-162.4144, 8.6692) -> (-162.809, 8.6577)
  line L1495 (-162.809, 8.6577) -> (-163.2034, 8.677)
  line L1496 (-163.2034, 8.677) -> (-163.6347, 8.743)
  line L1497 (-163.6347, 8.743) -> (-164.0589, 8.845)
  line L1498 (-164.0589, 8.845) -> (-164.453, 8.9915)
  line L1499 (-164.453, 8.9915) -> (-164.8284, 9.1809)
  line L1500 (-164.8284, 9.1809) -> (-165.1526, 9.4036)
  line L1501 (-165.1526, 9.4036) -> (-165.4339, 9.6653)
  line L1502 (-165.4339, 9.6653) -> (-165.6683, 9.9661)
  line L1503 (-165.6683, 9.9661) -> (-165.8558, 10.2981)
  line L1504 (-165.8558, 10.2981) -> (-165.9925, 10.6614)
  line L1505 (-165.9925, 10.6614) -> (-166.0706, 11.0481)
  line L1506 (-166.0706, 11.0481) -> (-166.0979, 11.4661)
  line L1507 (-166.0979, 11.4661) -> (-166.0823, 11.7473)
  line L1508 (-168.5511, -6.0847) -> (-168.4904, -5.6417)
  line L1509 (-168.4904, -5.6417) -> (-168.3909, -5.2058)
  line L1510 (-168.3909, -5.2058) -> (-168.2503, -4.8113)
  line L1511 (-168.2503, -4.8113) -> (-168.0706, -4.4558)
  line L1512 (-168.0706, -4.4558) -> (-167.8519, -4.1394)
  line L1513 (-167.8519, -4.1394) -> (-167.5979, -3.8699)
  line L1514 (-167.5979, -3.8699) -> (-167.305, -3.6433)
  line L1515 (-167.305, -3.6433) -> (-166.9847, -3.4636)
  line L1516 (-166.9847, -3.4636) -> (-166.6409, -3.3308)
  line L1517 (-166.6409, -3.3308) -> (-166.2776, -3.2449)
  line L1518 (-166.2776, -3.2449) -> (-165.8948, -3.2058)
  line L1519 (-165.8948, -3.2058) -> (-165.8089, -4.3386)
  line L1520 (-165.8089, -4.3386) -> (-166.0447, -4.3708)
  line L1521 (-166.0447, -4.3708) -> (-166.2745, -4.4296)
  line L1522 (-166.2745, -4.4296) -> (-166.4961, -4.5141)
  line L1523 (-166.4961, -4.5141) -> (-166.7073, -4.6238)
  line L1524 (-166.7073, -4.6238) -> (-166.9549, -4.8152)
  line L1525 (-166.9549, -4.8152) -> (-167.1594, -5.0484)
  line L1526 (-167.1594, -5.0484) -> (-167.3155, -5.3164)
  line L1527 (-167.3155, -5.3164) -> (-167.4183, -5.6121)
  line L1528 (-167.4183, -5.6121) -> (-167.5064, -6.116)
  line L1529 (-167.5064, -6.116) -> (-167.5278, -6.6249)
  line L1530 (-167.5278, -6.6249) -> (-167.4828, -7.1323)
  line L1531 (-167.4828, -7.1323) -> (-167.3714, -7.6316)
  line L1532 (-167.3714, -7.6316) -> (-167.2492, -7.9121)
  line L1533 (-167.2492, -7.9121) -> (-167.0715, -8.1567)
  line L1534 (-167.0715, -8.1567) -> (-166.8455, -8.3575)
  line L1535 (-166.8455, -8.3575) -> (-166.5784, -8.5066)
  line L1536 (-166.5784, -8.5066) -> (-166.3165, -8.5701)
  line L1537 (-166.3165, -8.5701) -> (-166.0507, -8.5688)
  line L1538 (-166.0507, -8.5688) -> (-165.793, -8.5042)
  line L1539 (-165.793, -8.5042) -> (-165.555, -8.3777)
  line L1540 (-165.555, -8.3777) -> (-165.3909, -8.2293)
  line L1541 (-165.3909, -8.2293) -> (-165.2056, -7.9325)
  line L1542 (-165.2056, -7.9325) -> (-165.0745, -7.6082)
  line L1543 (-165.0745, -7.6082) -> (-164.851, -6.8582)
  line L1544 (-164.851, -6.8582) -> (-164.6722, -6.0964)
  line L1545 (-164.6722, -6.0964) -> (-164.4812, -5.3454)
  line L1546 (-164.4812, -5.3454) -> (-164.2425, -4.6082)
  line L1547 (-164.2425, -4.6082) -> (-164.18, -4.4597)
  line L1548 (-164.18, -4.4597) -> (-163.9886, -4.0964)
  line L1549 (-163.9886, -4.0964) -> (-163.7737, -3.7839)
  line L1550 (-163.7737, -3.7839) -> (-163.5315, -3.5183)
  line L1551 (-163.5315, -3.5183) -> (-163.2698, -3.3074)
  line L1552 (-163.2698, -3.3074) -> (-162.9808, -3.1433)
  line L1553 (-162.9808, -3.1433) -> (-162.6761, -3.03)
  line L1554 (-162.6761, -3.03) -> (-162.3396, -2.9591)
  line L1555 (-162.3396, -2.9591) -> (-161.9964, -2.9363)
  line L1556 (-161.9964, -2.9363) -> (-161.6448, -2.9597)
  line L1557 (-161.6448, -2.9597) -> (-161.3011, -3.0378)
  line L1558 (-161.3011, -3.0378) -> (-160.9656, -3.1702)
  line L1559 (-160.9656, -3.1702) -> (-160.6487, -3.3425)
  line L1560 (-160.6487, -3.3425) -> (-160.3519, -3.573)
  line L1561 (-160.3519, -3.573) -> (-160.0901, -3.8425)
  line L1562 (-160.0901, -3.8425) -> (-159.8597, -4.1589)
  line L1563 (-159.8597, -4.1589) -> (-159.6646, -4.5261)
  line L1564 (-159.6646, -4.5261) -> (-159.512, -4.9128)
  line L1565 (-159.512, -4.9128) -> (-159.4026, -5.3347)
  line L1566 (-159.4026, -5.3347) -> (-159.3231, -6.0229)
  line L1567 (-159.3231, -6.0229) -> (-159.3276, -6.7131)
  line L1568 (-159.3276, -6.7131) -> (-159.4154, -7.3977)
  line L1569 (-159.4154, -7.3977) -> (-159.5862, -8.0691)
  line L1570 (-159.5862, -8.0691) -> (-159.7527, -8.4638)
  line L1571 (-159.7527, -8.4638) -> (-159.9736, -8.8283)
  line L1572 (-159.9736, -8.8283) -> (-160.2449, -9.1569)
  line L1573 (-160.2449, -9.1569) -> (-160.5628, -9.4441)
  line L1574 (-160.5628, -9.4441) -> (-160.7347, -9.5652)
  line L1575 (-160.7347, -9.5652) -> (-161.1019, -9.7722)
  line L1576 (-161.1019, -9.7722) -> (-161.4925, -9.9246)
  line L1577 (-161.4925, -9.9246) -> (-161.9065, -10.0183)
  line L1578 (-161.9065, -10.0183) -> (-162.344, -10.0574)
  line L1579 (-162.344, -10.0574) -> (-162.4417, -8.9402)
  line L1580 (-162.4417, -8.9402) -> (-162.2167, -8.911)
  line L1581 (-162.2167, -8.911) -> (-161.9957, -8.8619)
  line L1582 (-161.9957, -8.8619) -> (-161.7799, -8.7934)
  line L1583 (-161.7799, -8.7934) -> (-161.5706, -8.7058)
  line L1584 (-161.5706, -8.7058) -> (-161.3928, -8.6095)
  line L1585 (-161.3928, -8.6095) -> (-161.2288, -8.4924)
  line L1586 (-161.2288, -8.4924) -> (-161.0804, -8.3561)
  line L1587 (-161.0804, -8.3561) -> (-160.9495, -8.2019)
  line L1588 (-160.9495, -8.2019) -> (-160.7742, -7.9297)
  line L1589 (-160.7742, -7.9297) -> (-160.631, -7.6405)
  line L1590 (-160.631, -7.6405) -> (-160.5211, -7.337)
  line L1591 (-160.5211, -7.337) -> (-160.4456, -7.0222)
  line L1592 (-160.4456, -7.0222) -> (-160.3892, -6.6091)
  line L1593 (-160.3892, -6.6091) -> (-160.3783, -6.1935)
  line L1594 (-160.3783, -6.1935) -> (-160.4128, -5.7792)
  line L1595 (-160.4128, -5.7792) -> (-160.4925, -5.3699)
  line L1596 (-160.4925, -5.3699) -> (-160.5679, -5.1253)
  line L1597 (-160.5679, -5.1253) -> (-160.6727, -4.893)
  line L1598 (-160.6727, -4.893) -> (-160.8056, -4.6754)
  line L1599 (-160.8056, -4.6754) -> (-160.9651, -4.4753)
  line L1600 (-160.9651, -4.4753) -> (-161.101, -4.3521)
  line L1601 (-161.101, -4.3521) -> (-161.2506, -4.2507)
  line L1602 (-161.2506, -4.2507) -> (-161.4114, -4.1719)
  line L1603 (-161.4114, -4.1719) -> (-161.5809, -4.1164)
  line L1604 (-161.5809, -4.1164) -> (-161.7564, -4.0847)
  line L1605 (-161.7564, -4.0847) -> (-161.9353, -4.0775)
  line L1606 (-161.9353, -4.0775) -> (-162.1151, -4.0955)
  line L1607 (-162.1151, -4.0955) -> (-162.2933, -4.1394)
  line L1608 (-162.2933, -4.1394) -> (-162.4321, -4.1946)
  line L1609 (-162.4321, -4.1946) -> (-162.5615, -4.2678)
  line L1610 (-162.5615, -4.2678) -> (-162.6799, -4.3579)
  line L1611 (-162.6799, -4.3579) -> (-162.7854, -4.4636)
  line L1612 (-162.7854, -4.4636) -> (-162.9147, -4.6404)
  line L1613 (-162.9147, -4.6404) -> (-163.0272, -4.8277)
  line L1614 (-163.0272, -4.8277) -> (-163.1223, -5.0244)
  line L1615 (-163.1223, -5.0244) -> (-163.1995, -5.2292)
  line L1616 (-163.1995, -5.2292) -> (-163.4527, -6.1193)
  line L1617 (-163.4527, -6.1193) -> (-163.6722, -7.0183)
  line L1618 (-163.6722, -7.0183) -> (-163.8551, -7.6732)
  line L1619 (-163.8551, -7.6732) -> (-164.0901, -8.3113)
  line L1620 (-164.0901, -8.3113) -> (-164.2871, -8.674)
  line L1621 (-164.2871, -8.674) -> (-164.5315, -9.0066)
  line L1622 (-164.5315, -9.0066) -> (-164.8583, -9.3108)
  line L1623 (-164.8583, -9.3108) -> (-165.2384, -9.5349)
  line L1624 (-165.2384, -9.5349) -> (-165.6577, -9.6727)
  line L1625 (-165.6577, -9.6727) -> (-166.1019, -9.7175)
  line L1626 (-166.1019, -9.7175) -> (-166.4378, -9.6941)
  line L1627 (-166.4378, -9.6941) -> (-166.7611, -9.6189)
  line L1628 (-166.7611, -9.6189) -> (-167.0706, -9.4988)
  line L1629 (-167.0706, -9.4988) -> (-167.3714, -9.3308)
  line L1630 (-167.3714, -9.3308) -> (-167.6487, -9.116)
  line L1631 (-167.6487, -9.116) -> (-167.887, -8.8582)
  line L1632 (-167.887, -8.8582) -> (-168.094, -8.5574)
  line L1633 (-168.094, -8.5574) -> (-168.2686, -8.2034)
  line L1634 (-168.2686, -8.2034) -> (-168.3987, -7.8308)
  line L1635 (-168.3987, -7.8308) -> (-168.4746, -7.5194)
  line L1636 (-168.4746, -7.5194) -> (-168.5286, -7.204)
  line L1637 (-168.5286, -7.204) -> (-168.5607, -6.8855)
  line L1638 (-168.5607, -6.8855) -> (-168.5706, -6.5652)
  line L1639 (-168.5706, -6.5652) -> (-168.5511, -6.0847)
  line L1640 (-162.3206, -34.5886) -> (-161.7142, -34.6113)
  line L1641 (-161.7142, -34.6113) -> (-161.1136, -34.698)
  line L1642 (-161.1136, -34.698) -> (-160.8193, -34.7701)
  line L1643 (-160.8193, -34.7701) -> (-160.5389, -34.8813)
  line L1644 (-160.5389, -34.8813) -> (-160.2763, -35.0298)
  line L1645 (-160.2763, -35.0298) -> (-160.0354, -35.2136)
  line L1646 (-160.0354, -35.2136) -> (-159.8206, -35.448)
  line L1647 (-159.8206, -35.448) -> (-159.6409, -35.7214)
  line L1648 (-159.6409, -35.7214) -> (-159.4989, -36.0338)
  line L1649 (-159.4989, -36.0338) -> (-159.3987, -36.3621)
  line L1650 (-159.3987, -36.3621) -> (-159.3357, -36.7474)
  line L1651 (-159.3357, -36.7474) -> (-159.3167, -37.1362)
  line L1652 (-159.3167, -37.1362) -> (-159.3416, -37.5246)
  line L1653 (-159.3416, -37.5246) -> (-159.4104, -37.9089)
  line L1654 (-159.4104, -37.9089) -> (-159.4998, -38.1889)
  line L1655 (-159.4998, -38.1889) -> (-159.6281, -38.4516)
  line L1656 (-159.6281, -38.4516) -> (-159.7931, -38.693)
  line L1657 (-159.7931, -38.693) -> (-159.9925, -38.9089)
  line L1658 (-159.9925, -38.9089) -> (-160.182, -39.0608)
  line L1659 (-160.182, -39.0608) -> (-160.3873, -39.189)
  line L1660 (-160.3873, -39.189) -> (-160.6061, -39.2924)
  line L1661 (-160.6061, -39.2924) -> (-160.8362, -39.3699)
  line L1662 (-160.8362, -39.3699) -> (-161.1242, -39.4404)
  line L1663 (-161.1242, -39.4404) -> (-161.4165, -39.4875)
  line L1664 (-161.4165, -39.4875) -> (-161.7116, -39.5109)
  line L1665 (-161.7116, -39.5109) -> (-162.0081, -39.5105)
  line L1666 (-162.0081, -39.5105) -> (-162.1526, -38.4402)
  line L1667 (-162.1526, -38.4402) -> (-161.8916, -38.4271)
  line L1668 (-161.8916, -38.4271) -> (-161.6327, -38.3946)
  line L1669 (-161.6327, -38.3946) -> (-161.3769, -38.3429)
  line L1670 (-161.3769, -38.3429) -> (-161.1253, -38.2722)
  line L1671 (-161.1253, -38.2722) -> (-160.9271, -38.1835)
  line L1672 (-160.9271, -38.1835) -> (-160.7503, -38.0574)
  line L1673 (-160.7503, -38.0574) -> (-160.5862, -37.8699)
  line L1674 (-160.5862, -37.8699) -> (-160.4651, -37.6511)
  line L1675 (-160.4651, -37.6511) -> (-160.3948, -37.3972)
  line L1676 (-160.3948, -37.3972) -> (-160.3714, -37.1121)
  line L1677 (-160.3714, -37.1121) -> (-160.3807, -36.9099)
  line L1678 (-160.3807, -36.9099) -> (-160.4189, -36.7122)
  line L1679 (-160.4189, -36.7122) -> (-160.4851, -36.5221)
  line L1680 (-160.4851, -36.5221) -> (-160.5784, -36.3425)
  line L1681 (-160.5784, -36.3425) -> (-160.6855, -36.1953)
  line L1682 (-160.6855, -36.1953) -> (-160.8159, -36.0702)
  line L1683 (-160.8159, -36.0702) -> (-160.9662, -35.9699)
  line L1684 (-160.9662, -35.9699) -> (-161.1331, -35.8972)
  line L1685 (-161.1331, -35.8972) -> (-161.5099, -35.8131)
  line L1686 (-161.5099, -35.8131) -> (-161.8948, -35.7839)
  line L1687 (-161.8948, -35.7839) -> (-162.2503, -35.7761)
  line L1688 (-162.2503, -35.7761) -> (-168.4183, -35.7761)
  line L1689 (-168.4183, -35.7761) -> (-168.4183, -34.5886)
  line L1690 (-168.4183, -34.5886) -> (-162.3206, -34.5886)
  line L1691 (-166.0823, 5.0364) -> (-166.0465, 5.337)
  line L1692 (-166.0465, 5.337) -> (-165.9797, 5.6296)
  line L1693 (-165.9797, 5.6296) -> (-165.883, 5.9121)
  line L1694 (-165.883, 5.9121) -> (-165.7576, 6.1822)
  line L1695 (-165.7576, 6.1822) -> (-165.6047, 6.4378)
  line L1696 (-165.6047, 6.4378) -> (-165.4254, 6.6766)
  line L1697 (-165.4254, 6.6766) -> (-165.2209, 6.8964)
  line L1698 (-165.2209, 6.8964) -> (-164.9925, 7.095)
  line L1699 (-164.9925, 7.095) -> (-164.7331, 7.2704)
  line L1700 (-164.7331, 7.2704) -> (-164.4576, 7.4175)
  line L1701 (-164.4576, 7.4175) -> (-164.1683, 7.5351)
  line L1702 (-164.1683, 7.5351) -> (-163.8675, 7.6223)
  line L1703 (-163.8675, 7.6223) -> (-163.3887, 7.7034)
  line L1704 (-163.3887, 7.7034) -> (-162.9056, 7.7416)
  line L1705 (-162.9056, 7.7416) -> (-162.421, 7.7367)
  line L1706 (-162.421, 7.7367) -> (-161.9378, 7.6887)
  line L1707 (-161.9378, 7.6887) -> (-161.6517, 7.6453)